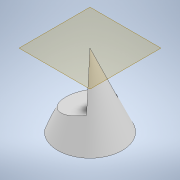
# Autodesk Inventor part: Деталь4
Saved by Autodesk Inventor 2021.2 (Build 252289000, 289)
## iProperties
Created: 2023-10-05
Part Number: Деталь4
Material: Типовые
Document SubType Name: Modeling
Designer: User
Density: 1 g/cm^3
Appearance: По умолчанию
Author: User
Autodesk Inventor part; units mm, degrees
ref_plane "YZ Plane" through (0, 0, 0) normal (1, 0, 0) x (0, 1, 0)
ref_plane "XY Plane" through (0, 0, 0) normal (0, 0, 1) x (1, 0, 0)
sketch "Эскиз1" plane through (0, 0, 0) normal (0, 1, 0) x (-1, 0, 0)
  circle A0 centre (0, 0) radius 40
  dimension "d0" = 80
  constraints: 1 centre point, 1 coincident
  measures "d0" diameter of A0
ref_plane "РабПлоскость1" through (0, 90, 0) normal (0, 1, 0) x (-1, 0, 0)
sketch "Эскиз2" plane through (0, 90, 0) normal (0, 1, 0) x (-1, 0, 0)
  point P0 (0, 0)
  point P1 (0, 0)
  constraints: 1 coincident
loft "Лофт1" add profiles "Эскиз1" section 1 point at (0, 90, 0)
sketch "Эскиз3" plane through (0, 0, 0) normal (0, 0, 1) x (1, 0, 0)
  line L0 (15, 0) -> (-30, 0)
  line L1 (-30, 0) -> (-30, 22.5)
  line L2 (15, 35) -> (-30, 22.5)
  line L3 (15, 35) -> (0, 90)
  line L4 (0, 90) -> (40, 0)
  line L5 (40, 0) -> (0, 90) projected
  line L6 (40, 0) -> (-40, 0) projected
  line L7 (15, 0) -> (40, 0)
  point P0 (0, 0)
  dimension "d6" = 45
  constraints: 12 end point, 1 collinear, 1 perpendicular, 1 point on line
  measures "d6" distance of L0.start L0.end
extrude "Выдавливание1" cut sketch "Эскиз3" against normal mid plane 90 keep common part
